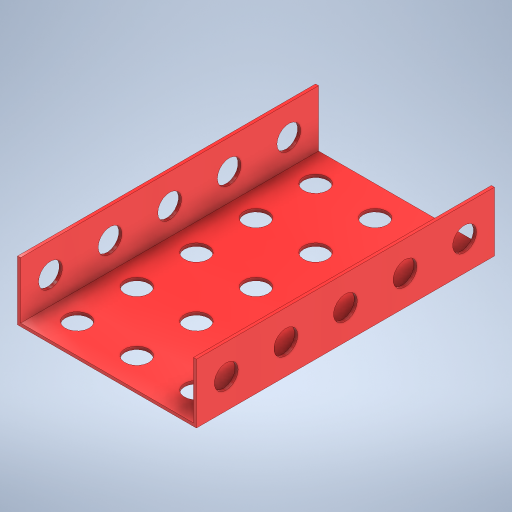
# Autodesk Inventor part: 1024 cervena
Saved by Autodesk Inventor 2024 (Build 280153000, 153)
## iProperties
Created: 2024-09-15
Part Number: 1024 cervena
Material: Všeobecné
Document SubType Name: Modeling
Designer: Student
Density: 1 g/cm^3
Appearance: Světle červená
Author: Student
Autodesk Inventor part; units mm, degrees
ref_plane "YZ Plane" through (0, 0, 0) normal (1, 0, 0) x (0, 1, 0)
ref_plane "XZ Plane" through (0, 0, 0) normal (0, 1, 0) x (-1, 0, 0)
ref_plane "XY Plane" through (0, 0, 0) normal (0, 0, 1) x (1, 0, 0)
sketch "Náčrt1" plane through (0, 0, 0) normal (0, 0, 1) x (1, 0, 0)
  line L0 (-14.5, 7.7937) -> (-14.5, -1.7063)
  line L1 (-14.5, -1.7063) -> (14.5, -1.7063)
  line L2 (14.5, -1.7063) -> (14.5, 7.7937)
  line L3 (14.5, 7.7937) -> (15, 7.7937)
  line L4 (15, 7.7937) -> (15, -2.2063)
  line L5 (15, -2.2063) -> (-15, -2.2063)
  line L6 (-15, -2.2063) -> (-15, 7.7937)
  line L7 (-15, 7.7937) -> (-14.5, 7.7937)
  point P0 (0, 0)
  point P1 (14.5, 3.0437)
  point P2 (-14.75, 7.7937)
  point P3 (14.75, 7.7937)
  dimension "d0" = 15
  dimension "d1" = 15
  dimension "d2" = 0.5
  dimension "d3" = 0.5
  dimension "d4" = 0.5
  dimension "d5" = 10
  dimension "d6" = 10
  constraints: 16 end point, 7 perpendicular, 3 midpoint, 1 vertical
  measures "d0" distance from line of L4 point (0, 0)
  measures "d1" distance from line of L6 point (0, 0)
  measures "d2" distance from line of L4 point (14.5, 3.044)
  measures "d3" distance between parallel lines of L6 L0
  measures "d4" distance between parallel lines of L5 L1
  measures "d5" distance from line of L5 point (-14.75, 7.794)
  measures "d6" vertical distance of L4.end point (14.75, 7.794)
extrude "Vysunutí1" add sketch "Náčrt1" along normal blind 50
sketch "Náčrt2" plane through (15, -2.2063, 0) normal (1, 0, 0) x (0, 0, -1)
  circle A0 centre (-5, 5) radius 2
  line L0 (0, 0) -> (0, 10) projected
  point P0 (0, 2.2063)
  point P1 (0, 5)
  dimension "d9" = 4
  dimension "d10" = 5
  constraints: 1 centre point, 1 midpoint
  measures "d9" diameter of A0
  measures "d10" distance of point (0, 5) A0.centre
extrude "Vysunutí2" cut sketch "Náčrt2" against normal through all
pattern_linear "Obdélníkové pole1" count 10 spacing 10 along (0, 0, 1) of "Vysunutí2"
sketch "Náčrt3" plane through (-14.5, -1.7063, 0) normal (0, 1, 0) x (1, 0, 0)
  circle A0 centre (4.5, -45) radius 2
  line L0 (29, -50) -> (0, -50) projected
  line L1 (-0.5, 0) -> (-0.5, -50) projected
  point P0 (14.5, 0)
  dimension "d16" = 4
  dimension "d17" = 5
  dimension "d18" = 5
  constraints: 1 centre point
  measures "d16" diameter of A0
  measures "d17" distance from line of L0 A0.centre
  measures "d18" distance from line of L1 A0.centre
extrude "Vysunutí3" cut sketch "Náčrt3" against normal through all
pattern_linear "Obdélníkové pole2" count 10 spacing 10 along (0, 0, -1) count 5 spacing 10 along (1, 0, 0) of "Vysunutí3"
